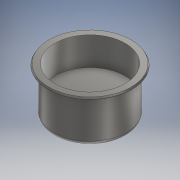
# Autodesk Inventor part: Bol
Saved by Autodesk Inventor 2017 (Build 210142000, 142)
## iProperties
Company: FABLAB Frenchmakers
Part Number: Bol
Material: Acier inoxydable
Document SubType Name: Modeling
Designer: FABLAB Frenchmakers
Density: 8 g/cm^3
Appearance: Semi-poli
Mass: 3809.82 g
Surface Area: 857.271 cm^2
Volume: 476.227 cm^3
Project: 1400-PopCorn Machine
Stock Number: 1400-01-01
Author: Adrien MARY
Autodesk Inventor part; units mm, degrees
ref_plane "YZ Plane" through (0, 0, 0) normal (1, 0, 0) x (0, 1, 0)
ref_plane "XZ Plane" through (0, 0, 0) normal (0, 1, 0) x (-1, 0, 0)
ref_plane "XY Plane" through (0, 0, 0) normal (0, 0, 1) x (1, 0, 0)
sketch "Esquisse1" plane through (0, 0, 0) normal (0, 0, 1) x (1, 0, 0)
  circle A0 centre (0, 0) radius 65
  dimension "d0" = 130
  constraints: 1 centre point, 1 coincident
  measures "d0" diameter of A0
extrude "Extrusion1" add sketch "Esquisse1" along normal blind 79
sketch "Esquisse2" plane through (0, 0, 79) normal (0, 0, 1) x (1, 0, 0)
  circle A0 centre (0, 0) radius 74.5
  dimension "d3" = 149
  constraints: 1 centre point, 1 coincident
  measures "d3" diameter of A0
extrude "Extrusion2" add sketch "Esquisse2" along normal blind 3
sketch "Esquisse3" plane through (0, 0, 82) normal (0, 0, 1) x (1, 0, 0)
  circle A0 centre (0, 0) radius 62.5
  dimension "d6" = 125
  constraints: 1 centre point, 1 coincident
  measures "d6" diameter of A0
extrude "Extrusion3" cut sketch "Esquisse3" against normal blind 50.5
fillet "Congé1" radius 8 1 edges at (-65, 0, 0)
fillet "Congé2" radius 4 1 edges at (-65, 0, 79)
chamfer "Chanfrein1" distance 1.5 angle 60 1 edges at (-74.5, 0, 82) measured on face at (-31.6394, -62.7681, 82)
equation "\"nombredor\" = 1.61803"
equation "\"pi\" = 3.141593"
